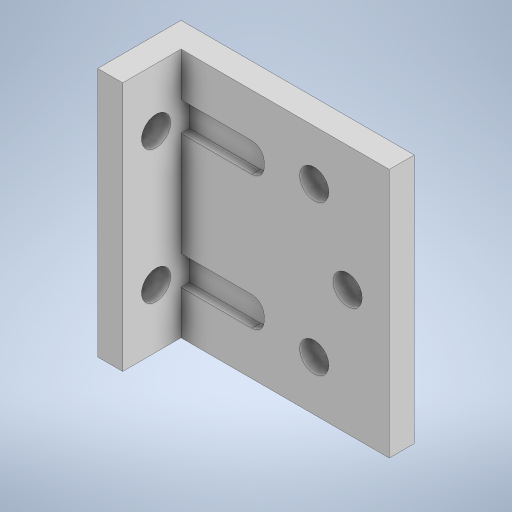
# Autodesk Inventor part: POUPLY_P4_V3
Saved by Autodesk Inventor 2024 (Build 280153000, 153)
## iProperties
Created: 2024-04-22
Part Number: POUPLY_P4_V3
Material: Generic
Document SubType Name: Modeling
Designer: luc4s
Density: 1 g/cm^3
Appearance: Default
Author: luc4s
Autodesk Inventor part; units mm, degrees
ref_plane "YZ Plane" through (0, 0, 0) normal (1, 0, 0) x (0, 1, 0)
ref_plane "XZ Plane" through (0, 0, 0) normal (0, 1, 0) x (-1, 0, 0)
ref_plane "XY Plane" through (0, 0, 0) normal (0, 0, 1) x (1, 0, 0)
sketch "Sketch1" plane through (0, 0, 0) normal (1, 0, 0) x (0, 1, 0)
  point P0 (0, 0)
sketch "Sketch2" plane through (0, 0, 0) normal (1, 0, 0) x (0, 1, 0)
  line L0 (15, 5) -> (-15, 5)
  line L1 (-15, 5) -> (-15, -5)
  line L2 (-15, -5) -> (15, -5)
  line L3 (15, -5) -> (15, 5)
  point P0 (0, 0)
  dimension "d0" = 10
  dimension "d1" = 30
  dimension "d2" = 15
  dimension "d3" = 5
  constraints: 8 end point, 2 parallel, 1 horizontal, 1 perpendicular
  measures "d0" distance of L2.end L0.start
  measures "d1" distance of L0.start L0.end
  measures "d2" horizontal distance of point (0, 0) L1.end
  measures "d3" vertical distance of point (0, 0) L0.start
extrude "Extrusion1" add sketch "Sketch2" along normal blind 3
sketch "Sketch3" plane through (3, 0, 0) normal (1, 0, 0) x (0, 0, -1)
  line L0 (5, -15) -> (5, 15) projected
  line L1 (-5, -15) -> (5, -15) projected
  line L2 (5, 15) -> (2, 15)
  line L3 (2, 15) -> (2, -15)
  line L4 (2, -15) -> (5, -15)
  line L5 (5, -15) -> (5, 15)
  dimension "d16" = 3
  constraints: 8 end point, 2 parallel, 1 horizontal, 1 perpendicular, 1 point on line
  measures "d16" distance of L0.end L2.end
sketch "Sketch4" plane through (0, 0, 0) normal (-1, 0, 0) x (0, 0, 1)
  circle A0 centre (1, 8) radius 1.75
  line L0 (5, 15) -> (5, -15) projected
  line L1 (-5, 15) -> (5, 15) projected
  dimension "d19" = 4
  dimension "d23" = 3.5
  dimension "d27" = 7
  constraints: 1 centre point
  measures "d19" distance from line of L0 A0.centre
  measures "d23" diameter of A0
  measures "d27" distance from line of L1 A0.centre
extrude "Extrusion4" add sketch "Sketch3" along normal blind 25
extrude "Extrusion5" cut sketch "Sketch4" against normal blind 25
mirror "Mirror1" about plane through (0, 0, 0) normal (0, 1, 0) of "Extrusion5"
sketch "Sketch5" plane through (3, -15, -2) normal (0, 0, 1) x (1, 0, 0)
  line L0 (0, 30) -> (0, 0) projected
  line L1 (0, 24.75) -> (10, 24.75)
  line L2 (10, 24.75) -> (10, 21.25)
  line L3 (10, 21.25) -> (0, 21.25)
  line L4 (0, 21.25) -> (0, 24.75)
  line L5 (0, 30) -> (25, 30) projected
  point P0 (-3, 15)
  point P1 (0, 21.25)
  dimension "d24" = 5.25
  dimension "d25" = 3.5
  dimension "d26" = 10
  constraints: 8 end point, 2 parallel, 1 horizontal, 1 perpendicular, 1 point on line
  measures "d24" distance from line of L5 L1.end
  measures "d25" distance of L1.end L2.end
  measures "d26" distance of L2.end L3.end
extrude "Extrusion6" cut sketch "Sketch5" against normal blind 1
fillet "Fillet2" radius 1.5 2 edges at (13, 9.75, -2.5) (13, 6.25, -2.5)
mirror "Mirror2" about plane through (0, 0, 0) normal (0, 1, 0) of "Extrusion6", "Fillet2"
sketch "Sketch6" plane through (3, -15, -2) normal (0, 0, 1) x (1, 0, 0)
  circle A0 centre (16, 24) radius 1.75
  circle A1 centre (20, 15) radius 1.75
  circle A2 centre (16, 6) radius 1.75
  line L0 (0, 30) -> (25, 30) projected
  line L1 (0, 0) -> (25, 0) projected
  line L2 (0, 30) -> (0, 0) projected
  line L3 (25, 30) -> (25, 0) projected
  point P0 (-3, 15)
  dimension "d31" = 3.5
  dimension "d32" = 3.5
  dimension "d33" = 3.5
  dimension "d34" = 6
  dimension "d35" = 6
  dimension "d36" = 15
  dimension "d40" = 9
  dimension "d41" = 5
  dimension "d42" = 9
  constraints: 3 centre point
  measures "d31" diameter of A1
  measures "d32" diameter of A0
  measures "d33" diameter of A2
  measures "d34" distance from line of L0 A0.centre
  measures "d35" distance from line of L1 A2.centre
  measures "d36" distance from line of L0 A1.centre
  measures "d40" distance from line of L3 A0.centre
  measures "d41" distance from line of L3 A1.centre
  measures "d42" distance from line of L3 A2.centre
extrude "Extrusion7" cut sketch "Sketch6" against normal blind 9 contours A0 | A1 | A2
body "Solid1"
